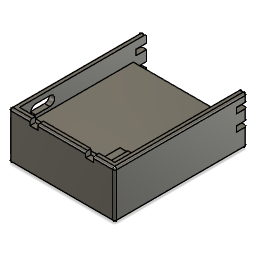
case_body (Autodesk Fusion 360 design; units mm, degrees)
Autodesk Fusion 360 part; units mm, degrees
note: some values were not read from the file. Set by a fixed rule: which sketch regions a step uses.
sketch "Sketch1" plane through (0, 0, 0) normal (0, 1, 0) x (1, 0, 0)
  line L0 (40, 0) -> (40, -50)
  line L1 (40, -50) -> (0, -50)
  line L2 (0, -50) -> (0, 0)
  line L3 (38, 0) -> (38, -6)
  line L4 (38, -6) -> (2, -6)
  line L5 (2, -6) -> (2, 0)
  line L6 (0, 0) -> (2, 0)
  line L7 (38, 0) -> (40, 0)
  dimension "d3" = 40
  dimension "d4" = 50
  dimension "d40" = 2
  dimension "d41" = 2
  dimension "d42" = 6
  constraint horizontal L6
  constraint vertical L0
  constraint horizontal L1
  constraint vertical L2
  constraint coincident L2.end L6.start
  constraint vertical L3
  constraint horizontal L4
  constraint vertical L5
  constraint collinear L6 L7
  measures "d3" distance of L2.end L0.start
  measures "d4" distance of L2.end L1.end
  measures "d40" distance of L2 L5
  measures "d41" distance of L0 L3
  measures "d42" distance of L5.end L4.end
extrude "Extrude1" add sketch "Sketch1" along normal blind 2
sketch "Sketch2" plane through (0, 2, 0) normal (0, 1, 0) x (-1, 0, 0)
  line L0 (0, 50) -> (-40, 50)
  line L1 (-40, 50) -> (-40, 0)
  line L2 (-2, 0) -> (0, 0)
  line L3 (0, 0) -> (0, 50)
  line L4 (0, 0) -> (-2, 0)
  line L5 (-2, 0) -> (-2, 48)
  line L6 (-1, 50) -> (0, 50)
  line L7 (0, 50) -> (0, 0)
  line L8 (-40, 50) -> (-1, 50)
  line L9 (-2, 48) -> (-38, 48)
  line L10 (-40, 44) -> (-40, 50)
  line L11 (-38, 0) -> (-38, 48)
  line L12 (-38, 6) -> (-2, 6)
  line L13 (-2, 6) -> (-2, 0)
  line L14 (-40, 0) -> (-38, 0)
  line L15 (-38, 0) -> (-38, 6)
  dimension "d18" = 2
  dimension "d19" = 2
  dimension "d20" = 2
  constraint horizontal L4
  constraint vertical L5
  constraint horizontal L6
  constraint vertical L7
  constraint coincident L0 L6.start
  constraint coincident L2.end L3.start
  constraint horizontal L8
  constraint horizontal L9
  constraint vertical L10
  constraint coincident L0.end L1.start
  constraint vertical L11
  measures "d18" distance of L8 L9
  measures "d19" distance of L5 L7
  measures "d20" distance of L10 L11
extrude "Extrude2" add sketch "Sketch2" along normal blind 16 contours L0 L1 L2 L3 L4 L5 L6 L7 L8 L9 L10 L11 L13 L14 L15
sketch "Sketch4" plane through (2, 0, 0) normal (1, 0, 0) x (0, 0, -1)
  line L0 (-48, 2) -> (-6, 2)
  line L1 (0, 0) -> (0, 18)
  line L2 (0, 18) -> (-48, 18)
  line L3 (-48, 18) -> (-48, 2)
  line L4 (-48, 11.3) -> (-5, 11.3)
  line L5 (-5, 11.3) -> (-5, 9.3)
  line L6 (-5, 9.3) -> (-48, 9.3)
  line L7 (-48, 9.3) -> (-48, 11.3)
  line L8 (-6, 0) -> (0, 0)
  line L9 (-6, 2) -> (-6, 0)
  dimension "d13" = 2
  dimension "d14" = 7.3
  dimension "d15" = 5
  constraint horizontal L4
  constraint vertical L5
  constraint horizontal L6
  constraint vertical L7
  constraint coincident L3 L4.start
  measures "d13" distance of L4 L6
  measures "d14" distance of L0 L6
  measures "d15" distance of L1 L5
extrude "Extrude4" add sketch "Sketch4" along normal up to surface (36 mm away) contours L3 L4 L5 L6 L7
sketch "Sketch5" plane through (2, 0, 0) normal (1, 0, 0) x (0, 0, -1)
  line L0 (-48, 11.3) -> (-5, 11.3)
  line L1 (-5, 11.3) -> (-5, 9.3)
  line L2 (-5, 9.3) -> (-48, 9.3)
  line L3 (-48, 9.3) -> (-48, 2)
  line L4 (-48, 2) -> (-6, 2)
  line L5 (0, 0) -> (0, 18)
  line L6 (0, 18) -> (-48, 18)
  line L7 (-48, 18) -> (-48, 11.3)
  line L8 (-43.7, 12.5) -> (-34.7, 12.5)
  line L9 (-34.7, 12.5) -> (-34.7, 16.1)
  line L10 (-34.7, 16.1) -> (-43.7, 16.1)
  line L11 (-43.7, 16.1) -> (-43.7, 12.5)
  line L12 (-6, 2) -> (-6, 0)
  line L13 (-6, 0) -> (0, 0)
  dimension "d21" = 4.3
  dimension "d43" = 1.2
  dimension "d68" = 1.9
  dimension "d69" = 9
  constraint horizontal L8
  constraint vertical L9
  constraint horizontal L10
  constraint vertical L11
  measures "d21" distance of L7 L11
  measures "d43" distance of L0 L8
  measures "d68" distance of L6 L10
  measures "d69" distance of L9.end L10.end
extrude "Extrude5" cut sketch "Sketch5" against normal up to surface (2 mm away) contours L8 L9 L10 L11
sketch "Sketch6" plane through (2, 0, 0) normal (1, 0, 0) x (0, 0, -1)
  line L0 (-34.7, 16.1) -> (-34.7, 12.5)
  line L1 (-34.7, 12.5) -> (-43.7, 12.5)
  line L2 (-43.7, 12.5) -> (-43.7, 16.1)
  line L3 (0, 18) -> (-48, 18)
  line L4 (-48, 18) -> (-48, 11.3)
  line L5 (-48, 11.3) -> (-5, 11.3)
  line L6 (-5, 11.3) -> (-5, 9.3)
  line L7 (-5, 9.3) -> (-48, 9.3)
  line L8 (-48, 9.3) -> (-48, 2)
  line L9 (-48, 2) -> (-6, 2)
  line L10 (0, 0) -> (0, 18)
  line L11 (-48, 15.3) -> (-46, 15.3)
  line L12 (-46, 15.3) -> (-46, 13.3)
  line L13 (-46, 13.3) -> (-48, 13.3)
  line L14 (-48, 13.3) -> (-48, 15.3)
  line L15 (-6, 2) -> (-6, 0)
  line L16 (-6, 0) -> (0, 0)
  line L17 (-43.7, 16.1) -> (-34.7, 16.1)
  dimension "d27" = 2
  dimension "d29" = 2
  dimension "d44" = 2
  constraint horizontal L11
  constraint vertical L12
  constraint horizontal L13
  constraint vertical L14
  constraint coincident L4 L13.end
  measures "d27" distance of L11.start L11.end
  measures "d29" distance of L11.start L13.end
  measures "d44" distance of L5 L13
extrude "Extrude6" add sketch "Sketch6" along normal up to surface (36 mm away) contours L4 L11 L12 L13 L14
sketch "Sketch7" plane through (0, 0, 46) normal (0, 0, -1) x (-1, 0, 0)
  line L0 (-2, 13.3) -> (-2, 15.3)
  line L1 (-2, 15.3) -> (-38, 15.3)
  line L2 (-38, 13.3) -> (-2, 13.3)
  line L3 (-38, 15.3) -> (-31, 15.3)
  line L4 (-31, 15.3) -> (-31, 13.3)
  line L5 (-31, 13.3) -> (-38, 13.3)
  line L6 (-38, 13.3) -> (-38, 15.3)
  line L7 (-38, 15.3) -> (-38, 13.3)
  dimension "d32" = 7
  constraint horizontal L3
  constraint vertical L4
  constraint horizontal L5
  constraint vertical L6
  constraint coincident L1.end L3.start
  constraint coincident L2 L5.end
  measures "d32" distance of L1.end L3.end
extrude "Extrude7" add sketch "Sketch7" along normal blind 7 contours L1 L2 L3 L4 L5 L6 L7
sketch "Sketch12" plane through (0, 15.3, 0) normal (0, 1, 0) x (-1, 0, 0)
  line L0 (-38, 48) -> (-38, 39)
  line L1 (-38, 39) -> (-31, 39)
  line L2 (-31, 39) -> (-31, 46)
  line L3 (-31, 46) -> (-2, 46)
  line L4 (-2, 46) -> (-2, 48)
  line L5 (-2, 48) -> (-38, 48)
  line L6 (-31, 39) -> (-34, 39)
  line L7 (-34, 39) -> (-34, 46)
  line L8 (-34, 46) -> (-31, 46)
  line L9 (-31, 46) -> (-31, 39)
  dimension "d78" = 3
  constraint horizontal L6
  constraint vertical L7
  constraint horizontal L8
  constraint vertical L9
  constraint coincident L1.end L2.start
  measures "d78" distance of L7.end L2.end
extrude "Extrude12" cut sketch "Sketch12" against normal blind 0.5 contours L1 L2 L6 L7 L8 L9
sketch "Sketch8" plane through (0, 0, 48) normal (0, 0, -1) x (-1, 0, 0)
  line L0 (-2, 13.3) -> (-38, 13.3)
  line L1 (-38, 13.3) -> (-38, 11.3)
  line L2 (-38, 11.3) -> (-2, 11.3)
  line L3 (-37.12, 13.3) -> (-35.12, 13.3)
  line L4 (-35.12, 13.3) -> (-35.12, 11.3)
  line L5 (-35.12, 11.3) -> (-37.12, 11.3)
  line L6 (-37.12, 11.3) -> (-37.12, 13.3)
  line L7 (-2, 11.3) -> (-2, 13.3)
  dimension "d35" = 2.88
  dimension "d36" = 2
  constraint horizontal L3
  constraint vertical L4
  constraint horizontal L5
  constraint vertical L6
  constraint coincident L2 L4.end
  constraint coincident L0 L3.end
  measures "d35" distance of L1 L4
  measures "d36" distance of L3.start L3.end
extrude "Extrude8" add sketch "Sketch8" along normal up to surface (9 mm away) contours L0 L2 L3 L4 L5 L6
sketch "Sketch10" plane through (0, 0, 0) normal (0, 0, -1) x (-1, 0, 0)
  line L0 (-40, 0) -> (-38, 0)
  line L1 (-38, 0) -> (-38, 18)
  line L2 (-38, 18) -> (-40, 18)
  line L3 (-40, 18) -> (-40, 0)
  line L4 (-40, 15) -> (-38, 15)
  line L5 (-38, 15) -> (-38, 12.9)
  line L6 (-38, 12.9) -> (-40, 12.9)
  line L7 (-40, 12.9) -> (-40, 15)
  line L8 (-40, 9) -> (-38, 9)
  line L9 (-38, 9) -> (-38, 6.9)
  line L10 (-38, 6.9) -> (-40, 6.9)
  line L11 (-40, 6.9) -> (-40, 9)
  dimension "d51" = 2.1
  dimension "d52" = 3
  dimension "d53" = 2.1
  dimension "d54" = 7
  constraint horizontal L4
  constraint vertical L5
  constraint horizontal L6
  constraint vertical L7
  constraint coincident L3 L4.start
  constraint horizontal L8
  constraint vertical L9
  constraint horizontal L10
  constraint vertical L11
  constraint midpoint L3 L8.start
  constraint coincident L1 L5.end
  constraint coincident L1 L9.end
  measures "d51" distance of L4.start L6.end
  measures "d52" distance of L2 L4
  measures "d53" distance of L8.start L10.end
extrude "Extrude10" cut sketch "Sketch10" against normal blind 4 contours L1 L3 L8 L9 L10 L11 | L1 L3 L4 L5 L6 L7
ref_plane "WorkPlane2" through (20, 9, 24) normal (-1, 0, 0) x (0, 0, 1)
mirror "Mirror1" about plane through (20, 9, 24) normal (-1, 0, 0) of "Extrude10"
sketch "Sketch11" plane through (0, 0, 48) normal (0, 0, -1) x (-1, 0, 0)
  line L0 (-38, 15.3) -> (-2, 15.3)
  line L1 (-2, 15.3) -> (-2, 18)
  line L2 (-2, 18) -> (-38, 18)
  line L3 (-38, 18) -> (-38, 15.3)
  line L4 (-32, 18) -> (-29, 18)
  line L5 (-29, 18) -> (-29, 16)
  line L6 (-29, 16) -> (-32, 16)
  line L7 (-32, 16) -> (-32, 18)
  line L8 (-11, 18) -> (-8, 18)
  line L9 (-8, 18) -> (-8, 16)
  line L10 (-8, 16) -> (-11, 16)
  line L11 (-11, 16) -> (-11, 18)
  dimension "d58" = 2
  dimension "d59" = 3
  dimension "d60" = 6
  dimension "d61" = 3
  dimension "d62" = 2
  dimension "d63" = 6
  constraint horizontal L4
  constraint vertical L5
  constraint horizontal L6
  constraint vertical L7
  constraint coincident L2 L4.start
  constraint horizontal L8
  constraint vertical L9
  constraint horizontal L10
  constraint vertical L11
  constraint coincident L2 L8.start
  measures "d58" distance of L4.start L6.end
  measures "d59" distance of L4.start L4.end
  measures "d60" distance of L3 L7
  measures "d61" distance of L8.start L8.end
  measures "d62" distance of L8.start L10.end
  measures "d63" distance of L1 L9
extrude "Extrude11" cut sketch "Sketch11" against normal up to surface (2 mm away) contours L2 L4 L5 L6 L7 | L2 L8 L9 L10 L11
sketch "Sketch13" plane through (0, 0, 0) normal (0, -1, 0) x (1, 0, 0)
  circle A0 centre (15, 23.5) radius 1.5
  circle A1 centre (15, 17.5) radius 1.5
  line L0 (20, 55.5) -> (20, 12.25)
  circle A2 centre (25, 23.5) radius 1.5
  circle A3 centre (25, 17.5) radius 1.5
  line L1 (2, 6) -> (38, 6)
  line L2 (38, 6) -> (38, 0)
  line L3 (38, 0) -> (40, 0)
  line L4 (40, 0) -> (40, 50)
  line L5 (40, 50) -> (0, 50)
  line L6 (0, 50) -> (0, 0)
  line L7 (0, 0) -> (2, 0)
  line L8 (2, 0) -> (2, 6)
  dimension "d81" = 3
  dimension "d83" = 3
  dimension "d84" = 6
  dimension "d85" = 26.5
  dimension "d86" = 15
  dimension "d87" = 20
  dimension "d88" = 20
  constraint symmetric A0 L0 A2
  constraint symmetric A1 L0 A3
  measures "d81" diameter of A0
  measures "d83" diameter of A1
  measures "d84" distance of A0.centre A1.centre
  measures "d85" distance of A0.centre L5
  measures "d86" distance of A0.centre L6
  measures "d87" distance of L0 L6
  measures "d88" distance of L0 L4
extrude "Extrude13" add sketch "Sketch13" along normal blind 0.5 contours A0 | A1 | A2 | A3
fillet "Fillet3" radius 1.5 4 edges at (13.6015, -0.5, 22.9576) (23.6015, -0.5, 22.9576) (23.6015, -0.5, 16.9576) (13.6015, -0.5, 16.9576)
fillet "Fillet1" radius 1.8 4 edges at (1, 12.5, 34.7) (1, 16.1, 34.7) (1, 12.5, 43.7) (1, 16.1, 43.7)
fillet "Fillet2" radius 0.75 12 edges at (40, 0, 25) (0, 0, 25) (20, 0, 50) (39, 0, 0) (1, 0, 0) (40, 18, 25) (0, 18, 25) (4, 18, 50) (20, 18, 50) (36, 18, 50) (40, 9, 50) (0, 9, 50)
fillet "Fillet2" radius 0.75 8 edges at (40, 3.45, 0) (40, 10.95, 0) (40, 16.5, 0) (0, 16.5, 0) (0, 10.95, 0) (0, 3.45, 0) (39, 18, 0) (1, 18, 0)
